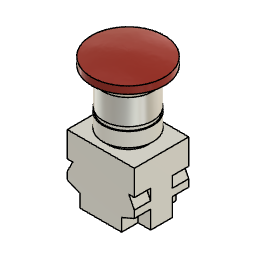
E-Stop (Autodesk Fusion 360 design; units mm, degrees)
Autodesk Fusion 360 part; units mm, degrees
sketch "Sketch1" plane through (0, 0, 0) normal (0, 1, 0) x (1, 0, 0)
  line L0 (0, 0) -> (37, 0)
  line L1 (37, 0) -> (37, -34)
  line L2 (37, -34) -> (0, -34)
  line L3 (0, -34) -> (0, 0)
  dimension "d1" = 37
  dimension "d2" = 34
  constraint horizontal L0
  constraint vertical L1
  constraint horizontal L2
  constraint vertical L3
  constraint coincident L0.start L3.end
  measures "d1" distance of L1.end L2.end
  measures "d2" distance of L0.end L1.end
extrude "Extrude1" add sketch "Sketch1" along normal blind 30
ref_plane "WorkPlane1" through (18.5, 15, 17) normal (0, -1, 0) x (-1, 0, 0)
sketch "Sketch3" plane through (18.5, 15, 17) normal (0, -1, 0) x (1, 0, 0)
  line L0 (18.5, 17) -> (-18.5, 17)
  line L1 (11, 17) -> (11, 19.7)
  line L2 (11, 19.7) -> (13.7, 19.7)
  line L3 (13.7, 19.7) -> (13.7, 27.5)
  line L4 (13.7, 27.5) -> (13.1, 27.5)
  line L5 (13.1, 27.5) -> (13.1, 29.7)
  line L6 (13.1, 29.7) -> (13.6, 29.7)
  line L7 (13.6, 29.7) -> (13.6, 43.7)
  line L8 (13.6, 43.7) -> (11.4, 43.7)
  line L9 (11.4, 43.7) -> (11.4, 49.7)
  line L10 (11.4, 49.7) -> (20, 49.7)
  line L11 (20, 49.7) -> (20, 53.7)
  arc A0 (20, 53.7) -> (0, 56) centre (-1.9407, -48.9821) ccw
  line L12 (0, 56) -> (0, 17)
  point P0 (-18.5, -17)
  dimension "d6" = 11
  dimension "d7" = 13.7
  dimension "d8" = 13.6
  dimension "d9" = 11.4
  dimension "d10" = 20
  dimension "d11" = 73
  dimension "d12" = 4
  dimension "d13" = 6
  dimension "d14" = 14
  dimension "d15" = 2.2
  dimension "d16" = 7.8
  dimension "d17" = 12.3
  dimension "d18" = 105
  dimension "d19" = 0.5
  constraint coincident L0 L1.start
  constraint perpendicular L0 L1
  constraint perpendicular L1 L2
  constraint perpendicular L2 L3
  constraint perpendicular L3 L4
  constraint perpendicular L4 L5
  constraint perpendicular L5 L6
  constraint perpendicular L6 L7
  constraint perpendicular L7 L8
  constraint perpendicular L8 L9
  constraint perpendicular L9 L10
  constraint perpendicular L10 L11
  constraint midpoint L0 L12.end
  constraint vertical L12
  measures "d6" distance of L1.start L12.end
  measures "d7" horizontal distance of L2.end L12.end
  measures "d8" horizontal distance of L6.end L12.end
  measures "d9" horizontal distance of L8.end L12.end
  measures "d10" horizontal distance of L10.end L12.end
  measures "d11" vertical distance of A0.end P0
  measures "d12" distance of L10.end L11.end
  measures "d13" distance of L8.end L9.end
  measures "d14" distance of L6.end L7.end
  measures "d15" distance of L4.end L5.end
  measures "d16" distance of L2.end L3.end
  measures "d17" vertical distance of L7.end A0.end
  measures "d18" radius of A0
  measures "d19" distance of L5.end L6.end
revolve "Revolve1" add sketch "Sketch3" angle 360 about axis through (18.5, 15, 73) along (0, 0, -1)
sketch "Sketch4" plane through (0, 0, 0) normal (0, -1, 0) x (1, 0, 0)
  line L0 (37, 34) -> (0, 34)
  line L1 (0, 34) -> (0, 0)
  line L2 (0, 0) -> (37, 0)
  line L3 (37, 0) -> (37, 34)
  line L4 (0, 20) -> (3, 20)
  line L5 (3, 20) -> (0, 14)
  line L6 (0, 10) -> (7, 7)
  line L7 (7, 7) -> (7, 0)
  dimension "d21" = 14
  dimension "d22" = 3
  dimension "d23" = 6
  dimension "d24" = 10
  dimension "d25" = 7
  dimension "d26" = 7
  constraint coincident L1 L4.start
  constraint perpendicular L1 L4
  constraint coincident L1 L5.end
  constraint coincident L1 L6.start
  constraint coincident L2 L7.end
  constraint perpendicular L2 L7
  measures "d21" distance of L0.end L4.start
  measures "d22" distance of L4.start L4.end
  measures "d23" distance of L4.start L5.end
  measures "d24" distance of L1.end L6.start
  measures "d25" distance of L1.end L7.end
  measures "d26" distance of L6.end L7.end
extrude "Extrude2" cut sketch "Sketch4" against normal blind 9 contours L1 L4 L5 | L1 L2 L6 L7
mirror "Mirror1" about plane through (18.5, 15, 17) normal (0, -1, 0) of "Extrude2"
ref_plane "WorkPlane3" through (18.5, 15, 17) normal (-1, 0, 0) x (0, 0, 1)
mirror "Mirror2" about plane through (18.5, 15, 17) normal (-1, 0, 0) of "Extrude2"
mirror "Mirror3" about plane through (18.5, 15, 17) normal (-1, 0, 0) of "Mirror1"
equation "d6 = ( 22 / 2 ) * 1 mm"
equation "d7 = ( 27.4 / 2 ) * 1 mm"
equation "d8 = ( 27.2 / 2 ) * 1 mm"
equation "d9 = ( 22.8 / 2 ) * 1 mm"
equation "d32 = ( -37 / 2 ) * 1 mm"
